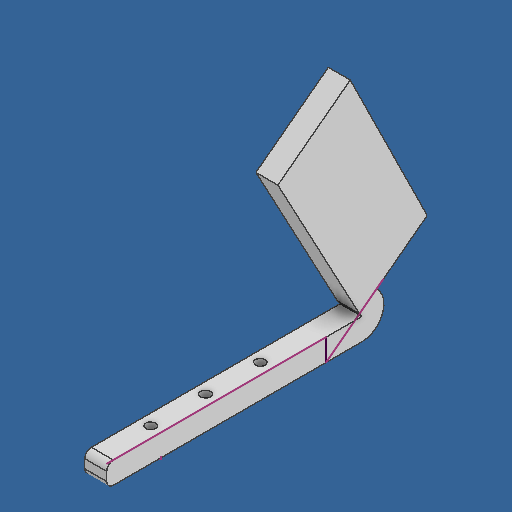
# Autodesk Inventor part: rod
Saved by Autodesk Inventor 2026.2 (Build 302298000, 298)
## iProperties
Created: 2025-12-16
Part Number: rod
Material: Generic
Document SubType Name: Modeling
Designer: Thoma
Density: 1 g/cm^3
Appearance: Default
Mass: 13.0768 g
Surface Area: 62.8747 cm^2
Volume: 13.0768 cm^3
Author: Thoma
Autodesk Inventor part; units mm, degrees
ref_plane "YZ Plane" through (0, 0, 0) normal (1, 0, 0) x (0, 1, 0)
ref_plane "XZ Plane" through (0, 0, 0) normal (0, 1, 0) x (-1, 0, 0)
ref_plane "XY Plane" through (0, 0, 0) normal (0, 0, 1) x (1, 0, 0)
sketch "Sketch1" plane through (0, 0, 0) normal (0, 1, 0) x (-1, 0, 0)
  line L0 (2.325581, 24.418605) -> (-7.674419, 24.418605)
  line L1 (-7.674419, 24.418605) -> (-7.674419, -75.581395)
  line L2 (-7.674419, -75.581395) -> (2.325581, -75.581395)
  line L3 (2.325581, -75.581395) -> (2.325581, 24.418605)
  point P0 (0, 0)
  dimension "d2" = 100
  dimension "d3" = 10
  constraints: 8 end point, 2 parallel, 1 horizontal, 1 perpendicular
  measures "d2" distance of L2.end L0.start
  measures "d3" distance of L0.start L0.end
extrude "Extrusion1" add sketch "Sketch1" along normal blind 10
sketch "Sketch9" plane through (7.674419, 0, 24.418605) normal (1, 0, 0) x (0, 0, -1)
  line L0 (0, 10) -> (100, 10) projected
  line L1 (0, 0) -> (100, 0) projected
  line L2 (0, 10) -> (100, 10)
  line L3 (100, 10) -> (100, 0)
  line L4 (100, 0) -> (0, 0)
  line L5 (0, 0) -> (0, 10)
  point P0 (24.418605, 0)
  constraints: 8 end point, 2 parallel, 1 horizontal, 1 perpendicular
extrude "Extrusion8" cut sketch "Sketch9" against normal blind 5
sketch "Sketch10" plane through (2.674419, 0, 24.418605) normal (1, 0, 0) x (0, 0, -1)
  line L0 (100, 0) -> (100, 10) projected
  line L1 (100, 10) -> (126, 10)
  line L2 (126, 10) -> (126, 29.842)
  line L3 (126, 29.842) -> (100, 10)
  line L4 (126, 29.842) -> (126, 19.842)
  line L5 (126, 19.842) -> (100, 0)
  point P0 (24.418605, 0)
  dimension "d44" = 19.842
  dimension "d45" = 26
  dimension "d46" = 10
  constraints: 10 end point, 1 horizontal, 1 perpendicular, 1 point on line
  measures "d44" distance of L1.end L2.end
  measures "d45" distance of L0.end L1.end
  measures "d46" distance of L2.end L4.end
extrude "Extrusion9" add sketch "Sketch10" against normal blind 5 contours L0 L1 L5 | L3 L2 L5 L1
sketch "Sketch12" plane through (2.674419, 0, 24.418605) normal (1, 0, 0) x (0, 0, -1)
  line L0 (100, 0) -> (0, 0)
  line L1 (126, 29.842) -> (126, 19.842)
  line L2 (99.933064, 0) -> (126, 19.842)
  line L3 (126, 19.842) -> (126, 29.842)
  line L4 (126, 29.842) -> (99.933064, 10)
  line L5 (99.933064, 10) -> (99.933064, 0)
  point P0 (24.418605, 0)
  constraints: 8 end point, 3 equal length
extrude "Extrusion10" add sketch "Sketch12" along normal blind 5
sketch "Sketch13" plane through (2.674419, 0, 24.418605) normal (1, 0, 0) x (0, 0, -1)
  line L0 (100, 10) -> (0, 10) projected
  line L1 (100, 0) -> (0, 0) projected
  line L2 (0, 10) -> (100, 10)
  line L3 (100, 10) -> (100, 0)
  line L4 (100, 0) -> (0, 0)
  line L5 (0, 0) -> (0, 10)
  point P0 (24.418605, 0)
  constraints: 8 end point, 2 parallel, 1 horizontal, 1 perpendicular
extrude "Extrusion11" add sketch "Sketch13" along normal blind 5
sketch "Sketch2" plane through (0, 10, 0) normal (0, 1, 0) x (1, 0, 0)
  line L0 (-2.325581, -24.418605) -> (7.674419, -24.418605)
  line L1 (7.674419, -24.418605) -> (7.674419, 75.581395)
  line L2 (-2.325581, -24.418605) -> (7.674419, -24.418605)
  line L3 (2.674419, -24.418605) -> (2.674419, -14.418605)
  line L4 (2.674419, -14.418605) -> (2.674419, -4.418605)
  line L5 (2.674419, -4.418605) -> (2.674419, 10.581395)
  line L6 (2.674419, 10.581395) -> (2.674419, 25.581395)
  line L7 (7.674419, 75.581395) -> (-2.325581, 75.581395)
  line L8 (-2.325581, 75.581395) -> (7.674419, 75.581395)
  line L9 (2.674419, -24.418605) -> (2.674419, 25.581395)
  line L10 (2.674419, 25.581395) -> (7.674419, 25.581395)
  line L11 (2.674419, 25.581395) -> (-2.325581, 25.581395)
  line L12 (-2.325581, 75.581395) -> (-2.325581, -24.418605)
  line L13 (2.674419, 25.581395) -> (2.674419, 40.581395)
  line L14 (2.674419, 25.581395) -> (2.674419, 75.581395)
  line L15 (2.674419, 0.581395) -> (-2.325581, 0.581395)
  line L16 (2.674419, 0.581395) -> (7.674419, 0.581395)
  line L17 (2.674419, 50.581395) -> (-2.325581, 50.581395)
  line L18 (7.674419, 50.581395) -> (2.674419, 50.581395)
  circle A0 centre (2.674419, 0.581395) radius 2.25
  circle A1 centre (2.674419, 25.581395) radius 2.25
  circle A2 centre (2.674419, 50.581395) radius 2.25
  point P0 (0, 0)
  dimension "d28" = 4.5
  dimension "d29" = 4.5
  dimension "d30" = 4.5
  constraints: 30 end point, 6 midpoint, 6 point on line, 5 coincident, 5 vertical, 3 centre point, 2 collinear, 2 perpendicular, 1 horizontal
  measures "d28" diameter of A0
  measures "d29" diameter of A1
  measures "d30" diameter of A2
extrude "Extrusion2" cut sketch "Sketch2" against normal blind 10 contours A0 L5 L15 | L15 L5 A0 | A1 L13 L11 | L11 L6 A1 | L16 A0 L5 | L5 A0 L16 | L10 A1 L6 | L13 A1 L10 | A2 L14 L17 | L17 L14 A2 | L18 A2 L14 | L14 A2 L18
sketch "Sketch14" plane through (7.674419, 0, 24.418605) normal (1, 0, 0) x (0, 0, -1)
  line L0 (100, 10) -> (0, 10) projected
  line L1 (126, 19.842) -> (100, 0) projected
  line L2 (100, 10) -> (100, 0)
  point P0 (24.418605, 0)
  constraints: 2 end point, 1 vertical
sketch "Sketch16" plane through (7.674419, 0, 24.418605) normal (1, 0, 0) x (0, 0, -1)
  line L0 (100, 10) -> (126, 29.842)
  line L1 (100, 10) -> (112.896482, 19.842)
  line L2 (112.896482, 19.842) -> (113.514198, 20.313412)
  line L3 (113.514198, 20.313412) -> (118.329114, 14.004177)
  line L4 (117.711399, 13.532765) -> (112.884086, 19.858243)
  line L5 (117.711399, 13.532765) -> (118.329114, 14.004177)
  point P0 (24.418605, 0)
  dimension "d60" = 16.22295
  dimension "d61" = 0.77705
  constraints: 8 end point, 1 collinear, 1 parallel, 1 point on line
  measures "d60" distance of L0.start L1.end
  measures "d61" distance of L1.end L2.end
extrude "Extrusion13" add sketch "Sketch16" against normal blind 10
sketch "Sketch20" plane through (7.674419, 0, 24.418605) normal (1, 0, 0) x (0, 0, -1)
  line L0 (100, 10) -> (0, 10) projected
  line L1 (100, 10) -> (128, 10)
  line L2 (128, 10) -> (128, 0)
  line L3 (128, 0) -> (100, 0)
  line L4 (100, 0) -> (100, 10)
  line L5 (126, 29.842) -> (100, 10) projected
  line L6 (100, 10) -> (126, 10)
  line L7 (126, 10) -> (126, 29.842)
  line L8 (126, 29.842) -> (100, 29.842)
  line L9 (100, 29.842) -> (100, 10)
  point P0 (24.418605, 0)
  dimension "d77" = 28
  constraints: 16 end point, 4 parallel, 2 horizontal, 2 perpendicular
  measures "d77" distance of L2.end L3.end
extrude "Extrusion17" add sketch "Sketch20" against normal blind 10 contours L1 L2 L3 L4
sketch "Sketch21" plane through (7.674419, 0, 24.418605) normal (1, 0, 0) x (0, 0, -1)
  line L0 (128, 0) -> (128, 10)
  line L1 (128, 0) -> (151.87052, 18.170101)
  line L2 (113.070317, 10) -> (126, 19.842)
  line L3 (128, 10) -> (151.239467, 27.689747)
  line L4 (151.87052, 18.170101) -> (151.87052, 28.170101)
  line L5 (151.87052, 28.170101) -> (151.239467, 27.689747)
  line L6 (100, 10) -> (0, 10)
  line L7 (126, 29.842) -> (100, 29.842)
  line L8 (100, 29.842) -> (100, 10)
  line L9 (100, 10) -> (126, 10)
  line L10 (126, 10) -> (126, 29.842)
  point P0 (24.418605, 0)
  constraints: 16 end point, 4 parallel, 1 collinear, 1 horizontal, 1 perpendicular, 1 vertical
extrude "Extrusion18" add sketch "Sketch21" against normal blind 10 contours L0 L3 L5 L4 L1
sketch "Sketch22" plane through (7.674419, 0, 24.418605) normal (1, 0, 0) x (0, 0, -1)
  line L0 (100, 10) -> (126, 29.842) projected
  line L1 (100, 10) -> (0, 10) projected
  line L2 (126, 29.842) -> (100, 29.842)
  line L3 (100, 29.842) -> (100, 10)
  line L4 (100, 10) -> (126, 10)
  line L5 (126, 10) -> (126, 29.842)
  point P0 (24.418605, 0)
  constraints: 8 end point, 2 parallel, 1 horizontal, 1 perpendicular
extrude "Extrusion19" cut sketch "Sketch22" against normal blind 10
sketch "Sketch23" plane through (7.674419, 0, 24.418605) normal (1, 0, 0) x (0, 0, -1)
  line L0 (151.87052, 18.170101) -> (128, 0)
  line L1 (141.891396, 10.57405) -> (136.99663, 17.004426)
  line L2 (128, 0) -> (151.87052, 18.170101)
  line L3 (128, 10) -> (151.87052, 28.170101)
  line L4 (137.071931, 16.905501) -> (151.87052, 28.170101)
  line L5 (151.87052, 28.170101) -> (151.87052, 18.170101)
  line L6 (141.891396, 10.57405) -> (151.87052, 18.170101)
  point P0 (24.418605, 0)
  point P1 (137.071931, 16.905501)
  constraints: 8 end point, 2 collinear, 2 point on line, 1 perpendicular, 1 vertical
extrude "Extrusion20" cut sketch "Sketch23" against normal blind 10
sketch "Sketch24" plane through (7.674419, 0, 24.418605) normal (1, 0, 0) x (0, 0, -1)
  line L0 (141.891396, 10.57405) -> (137.071931, 16.905501)
  line L1 (137.071931, 16.905501) -> (120.042183, 39.277911)
  line L2 (120.042183, 39.277911) -> (114.78111, 35.273213)
  line L3 (114.78111, 35.273213) -> (131.810859, 12.900804)
  line L4 (128, 10) -> (137.071931, 16.905501)
  line L5 (130.433663, 25.626361) -> (125.172591, 21.621663)
  point P0 (24.418605, 0)
  constraints: 8 end point, 3 perpendicular, 3 point on line, 1 collinear
extrude "Extrusion21" add sketch "Sketch24" against normal blind 10 contours L4 L3 L5 L1
sketch "Sketch25" plane through (7.674419, 0, 24.418605) normal (1, 0, 0) x (0, 0, -1)
  circle A0 centre (130.028114, 20.963065) radius 1.414214
  line L0 (128, 0) -> (141.891396, 10.57405)
  point P0 (24.418605, 0)
  dimension "d88" = 15.452
  constraints: 1 centre point
  measures "d88" distance from line of L0 A0.centre
extrude "Extrusion22" cut sketch "Sketch25" against normal blind 10
sketch "Sketch26" plane through (7.674419, 0, 24.418605) normal (1, 0, 0) x (0, 0, -1)
  line L0 (146.180534, 13.38523) -> (129.005429, 0.311641)
  line L1 (128, 0) -> (141.891396, 10.57405)
  line L2 (129.005429, 0.311641) -> (127.101128, -1.137903)
  line L3 (128, 0) -> (128.596019, 0)
  line L4 (128, 10) -> (141.733271, 10)
  point P0 (24.418605, 0)
  point P1 (137.592982, 6.848436)
  point P2 (141.137252, 10)
  dimension "d89" = 0.361
  constraints: 8 end point, 2 parallel, 2 point on line, 1 collinear, 1 horizontal, 1 midpoint
  measures "d89" distance from line of point (137.593, 6.848) L1
extrude "Extrusion23" add sketch "Sketch26" against normal blind 10
sketch "Sketch27" plane through (7.674419, 0, 24.418605) normal (1, 0, 0) x (0, 0, -1)
  line L0 (128.596019, 0) -> (141.733271, 10)
  line L1 (141.733271, 10) -> (143.644553, 11.454856)
  line L2 (141.733271, 10) -> (141.137252, 10)
  line L3 (141.733271, 10) -> (141.137252, 10)
  line L4 (141.137252, 10) -> (143.4259, 11.742106)
  line L5 (143.4259, 11.742106) -> (143.644553, 11.454856)
  line L6 (143.4259, 11.742106) -> (141.608381, 14.129826)
  line L7 (141.608381, 14.129826) -> (140.073877, 12.96177)
  line L8 (130.433663, 25.626361) -> (141.891396, 10.57405)
  line L9 (141.891396, 10.57405) -> (140.073877, 12.96177)
  line L10 (141.891396, 10.57405) -> (130.433663, 25.626361)
  point P0 (24.418605, 0)
  dimension "d92" = 2.402
  constraints: 14 end point, 4 perpendicular, 3 point on line, 2 collinear, 1 parallel
  measures "d92" distance of L0.end L1.end
extrude "Extrusion24" add sketch "Sketch27" against normal blind 10
sketch "Sketch28" plane through (7.674419, 0, 24.418605) normal (1, 0, 0) x (0, 0, -1)
  line L0 (129.774875, 26.828636) -> (140.680759, 12.501302)
  line L1 (140.073877, 12.96177) -> (130.433663, 25.626361)
  line L2 (130.433663, 25.626361) -> (130.595987, 25.749921)
  line L3 (140.073877, 12.96177) -> (141.608381, 14.129826)
  line L4 (140.073877, 12.96177) -> (140.2362, 13.08533)
  line L5 (140.073877, 12.96177) -> (130.433663, 25.626361)
  point P0 (24.418605, 0)
  dimension "d95" = 0.204
  constraints: 8 end point, 3 point on line, 1 collinear, 1 parallel, 1 perpendicular
  measures "d95" distance between parallel lines of L0 L1
extrude "Extrusion25" add sketch "Sketch28" against normal blind 10
sketch "Sketch29" plane through (7.674419, 0, 24.418605) normal (1, 0, 0) x (0, 0, -1)
  line L0 (130.595987, 25.749921) -> (140.2362, 13.08533)
  line L1 (130.595987, 25.749921) -> (115.000185, 13.878487)
  line L2 (143.644553, 11.454856) -> (128.596019, 0)
  line L3 (137.494115, 6.773179) -> (119.565826, 30.326023)
  line L4 (122.798086, 19.814204) -> (116.546182, 28.027488)
  circle A0 centre (116.546182, 28.027488) radius 3
  line L5 (116.546182, 28.027488) -> (116.546182, 10)
  line L6 (0, 10) -> (128, 10)
  line L7 (128, 10) -> (100, 10)
  line L8 (116.546182, 28.027488) -> (110.546182, 28.027488)
  line L9 (110.546182, 28.027488) -> (110.546182, 34.027488)
  line L10 (116.546182, 28.027488) -> (122.546182, 28.027488)
  line L11 (122.546182, 28.027488) -> (122.546182, 10)
  line L12 (110.546182, 34.027488) -> (122.546182, 34.027488)
  line L13 (122.546182, 34.027488) -> (122.546182, 10)
  line L14 (122.546182, 10) -> (110.546182, 10)
  line L15 (110.546182, 10) -> (110.546182, 34.027488)
  point P0 (24.418605, 0)
  point P1 (122.546182, 28.027488)
  point P2 (110.546182, 28.027488)
  point P3 (110.546182, 10)
  point P4 (122.546182, 10)
  dimension "d98" = 19.6
  dimension "d99" = 29.6
  dimension "d100" = 6
  dimension "d101" = 6
  dimension "d102" = 6
  dimension "d103" = 6
  constraints: 24 end point, 5 perpendicular, 3 horizontal, 3 parallel, 3 point on line, 2 vertical, 1 centre point, 1 coincident, 1 midpoint
  measures "d98" distance of L0.start L1.end
  measures "d99" distance of L3.start L3.end
  measures "d100" diameter of A0
  measures "d101" distance of L5.start L8.end
  measures "d102" distance of L8.end L9.end
  measures "d103" distance of L5.start L10.end
extrude "Extrusion26" add sketch "Sketch29" against normal blind 10 contours L11 L4 A0 L10 L3 | L3 L10 L11 | L11 L6 L5 L1 | L1 L5 A0 L4 L11 | L10 A0 L8 L9 L12 L13 | L5 L6 L15 L8 A0
sketch "Sketch30" plane through (7.674419, 0, 24.418605) normal (1, 0, 0) x (0, 0, -1)
  line L0 (122.546182, 34.027488) -> (122.546182, 10)
  line L1 (122.546182, 34.027488) -> (144, 34.027488)
  line L2 (144, 34.027488) -> (144, 0)
  line L3 (144, 0) -> (122.546182, 0)
  line L4 (122.546182, 0) -> (122.546182, 34.027488)
  point P0 (24.418605, 0)
  constraints: 8 end point, 2 parallel, 1 horizontal, 1 perpendicular
extrude "Extrusion27" cut sketch "Sketch30" against normal blind 10
sketch "Sketch31" plane through (7.674419, 0, 24.418605) normal (1, 0, 0) x (0, 0, -1)
  line L0 (110.546182, 34.027488) -> (110.546182, 10)
  line L1 (110.546182, 10) -> (113, 10)
  line L2 (110.546182, 10) -> (114, 10)
  line L3 (114, 10) -> (114, 17)
  line L4 (114, 17) -> (110.546182, 17)
  line L5 (110.546182, 17) -> (110.546182, 10)
  point P0 (24.418605, 0)
  constraints: 10 end point, 2 horizontal, 2 parallel, 1 perpendicular
extrude "Extrusion28" cut sketch "Sketch31" against normal blind 10
sketch "Sketch32" plane through (7.674419, 0, 24.418605) normal (1, 0, 0) x (0, 0, -1)
  line L0 (114, 17) -> (110.546182, 17)
  line L1 (114, 17) -> (114, 10)
  line L2 (110.546182, 17) -> (114, 10)
  line L3 (114, 10) -> (114, 17)
  line L4 (114, 17) -> (110.546182, 17)
  point P0 (24.418605, 0)
  constraints: 6 end point, 1 collinear, 1 perpendicular
extrude "Extrusion29" add sketch "Sketch32" against normal blind 10
sketch "Sketch33" plane through (7.674419, 0, 24.418605) normal (1, 0, 0) x (0, 0, -1)
  line L0 (100, 10.050951) -> (99.933064, 10)
  line L1 (100, 10.050951) -> (99.933064, 10)
  line L2 (99.933064, 10) -> (100, 10)
  line L3 (99.933064, 10) -> (100, 10)
  line L4 (100, 10) -> (100, 10.050951)
  line L5 (100, 10) -> (100, 10.050951)
  point P0 (24.418605, 0)
  constraints: 6 end point, 2 collinear, 1 perpendicular
extrude "Extrusion30" cut sketch "Sketch33" against normal blind 10
sketch "Sketch34" plane through (7.674419, 0, 24.418605) normal (1, 0, 0) x (0, 0, -1)
  line L0 (119.614525, 21.220993) -> (127.725416, 4.782304)
  line L1 (110.546182, 17) -> (114, 10)
  line L2 (127.725416, 4.782304) -> (130.085017, 0)
  line L3 (122.546182, 0) -> (0, 0)
  line L4 (116.504679, 0) -> (130.085017, 0)
  line L5 (127.725416, 4.782304) -> (130.085017, 0)
  line L6 (122.546182, 34.027488) -> (122.546182, 0)
  line L7 (122.546182, 15.279278) -> (122.546182, 0)
  point P0 (24.418605, 0)
  dimension "d114" = 10
  constraints: 10 end point, 3 point on line, 2 collinear, 1 parallel, 1 perpendicular
  measures "d114" distance between parallel lines of L0 L1
extrude "Extrusion31" add sketch "Sketch34" against normal blind 10
fillet "Fillet2" radius 2 1 edges at (2.6744, 0, -105.6664)
fillet "Fillet3" radius 3 6 edges at (2.6744, 15.2793, -98.1276) (2.6744, 34.0275, -98.1276) (2.6744, 34.0275, -86.1276) (2.6744, 17, -86.1276) (2.6744, 10, 24.4186) (2.6744, 0, 24.4186)
sketch "Sketch35" plane through (7.674419, 0, 24.418605) normal (1, 0, 0) x (0, 0, -1)
  arc A0 (110.546182, 17.699829) -> (110.855838, 16.372406) centre (113.546182, 17.699829) ccw
  line L0 (110.546182, 17.699829) -> (115.999721, 10.054757)
  line L1 (115.999721, 10.054757) -> (113.999721, 10.054757)
  line L2 (110.546182, 17.699829) -> (110.546182, 10.054757)
  line L3 (110.546182, 10.054757) -> (115.999721, 10.054757)
  line L4 (114, 10) -> (3, 10)
  line L5 (110.546182, 10.054757) -> (115.999721, 10.054757)
  point P0 (24.418605, 0)
  point P1 (3, 10)
  constraints: 10 end point, 1 collinear, 1 horizontal, 1 perpendicular, 1 vertical, 1 other
extrude "Extrusion32" cut sketch "Sketch35" against normal blind 10
sketch "Sketch36" plane through (7.674419, 0, 24.418605) normal (1, 0, 0) x (0, 0, -1)
  line L0 (107, 10) -> (116.657393, 10)
  line L1 (110.546182, 17.699829) -> (115.999721, 10.054757)
  line L2 (3, 0) -> (126.868013, 0)
  line L3 (126, 19.842105) -> (100, 0)
  line L4 (114.482105, 12.631671) -> (116.575951, 9.696402)
  line L5 (115.211679, 11.608913) -> (109.490162, 19.106074)
  line L6 (110.546182, 31.027488) -> (110.546182, 17.699829)
  line L7 (110.546182, 17.699829) -> (110.546182, 10)
  line L8 (110.546182, 10) -> (116.359382, 10)
  point P0 (24.418605, 0)
  point P1 (110.546182, 17.722323)
  dimension "d121" = 0.261
  constraints: 12 end point, 6 point on line, 2 perpendicular, 1 horizontal, 1 parallel
  measures "d121" distance between parallel lines of L4 L1
extrude "Extrusion33" cut sketch "Sketch36" against normal blind 10
fillet "Fillet5" radius 3 1 edges at (2.6744, 17.7223, -86.1276)
sketch "Sketch37" plane through (7.674419, 0, 24.418605) normal (1, 0, 0) x (0, 0, -1)
  line L0 (117.932308, 24.527287) -> (136.6505, 0)
  line L1 (111.161328, 16.91627) -> (115.211679, 11.608913)
  line L2 (126.868013, 0) -> (3, 0)
  line L3 (122.31822, 0) -> (151, 0)
  line L4 (122.56441, 18.457636) -> (122.56441, 0)
  line L5 (122, 19.197208) -> (122, 0)
  point P0 (24.418605, 0)
  dimension "d126" = 10
  constraints: 8 end point, 6 point on line, 2 perpendicular, 1 collinear, 1 parallel
  measures "d126" distance between parallel lines of L0 L1
extrude "Extrusion34" add sketch "Sketch37" against normal blind 10
fillet "Fillet6" radius 3 2 edges at (2.6744, 0, -112.2319) (2.6744, 18.4815, -98.1276)
sketch "Sketch38" plane through (7.674419, 0, 24.418605) normal (1, 0, 0) x (0, 0, -1)
  line L0 (116.359382, 10) -> (115.211679, 11.608913)
  circle A0 centre (116.359382, 10) radius 10
  line L1 (116.359382, 0) -> (138.255518, 0)
  line L2 (123.161328, 17.675467) -> (132.972064, 4.82002)
  line L3 (125.598358, 14.482118) -> (136.6505, 0)
  line L4 (122.546182, 31.027488) -> (122.546182, 19.495487)
  line L5 (122.546182, 23.627159) -> (122.546182, 15.627103)
  line L6 (127.492606, 12) -> (119.861027, 22)
  line L7 (122.546182, 18.376494) -> (125.877807, 14.010917)
  line L8 (132.972064, 4.82002) -> (123.161328, 17.675467)
  line L9 (122.546182, 18.376494) -> (122.546182, 19.495487)
  line L10 (136.6505, 0) -> (122.546182, 19.495487)
  point P0 (24.418605, 0)
  point P1 (124.308895, 16.066733)
  dimension "d130" = 20
  constraints: 14 end point, 6 point on line, 3 collinear, 2 horizontal, 2 parallel, 4 other
extrude "Extrusion35" cut sketch "Sketch38" against normal blind 10 contours A0 L7 L5 L6 L2 L3 L1 | L3 L2 L6 L5 L10
sketch "Sketch39" plane through (7.674419, 0, 24.418605) normal (1, 0, 0) x (0, 0, -1)
  point P0 (24.418605, 0)
sketch "Sketch41" plane through (7.674419, 0, 24.418605) normal (1, 0, 0) x (0, 0, -1)
  line L0 (111.161328, 16.91627) -> (115.211679, 11.608913)
  line L1 (115.211679, 11.608913) -> (123.086785, 17.618862)
  line L2 (123.086785, 17.618862) -> (124, 35)
  line L3 (124, 35) -> (108, 35)
  line L4 (108, 35) -> (109, 11.608913)
  line L5 (109, 11.608913) -> (115.211679, 11.608913)
  point P0 (24.418605, 0)
  constraints: 10 end point, 2 point on line, 1 perpendicular
extrude "Extrusion37" cut sketch "Sketch41" against normal blind 10
sketch "Sketch42" plane through (7.674419, 0, 24.418605) normal (1, 0, 0) x (0, 0, -1)
  line L0 (115.211679, 11.608913) -> (78, 81)
  line L1 (78, 81) -> (111, 106)
  line L2 (111, 106) -> (146.082916, 34.996214)
  line L3 (146.082916, 34.996214) -> (115.211679, 11.608913)
  point P0 (24.418605, 0)
  constraints: 8 end point, 1 parallel
extrude "Extrusion38" add sketch "Sketch42" against normal blind 10
equation "\"d0\" = d3"
body "Solid1"
